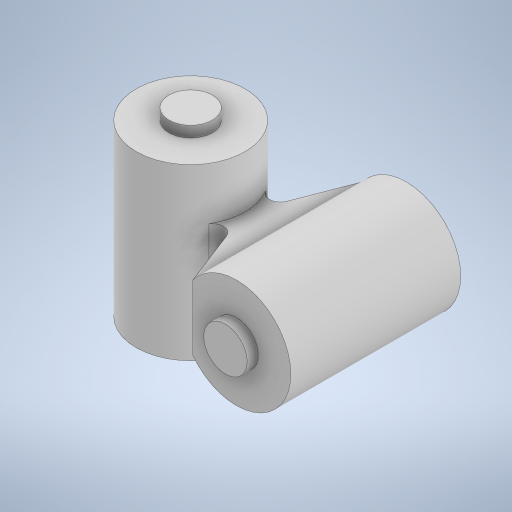
# Autodesk Inventor part: Arm 4 v0.1
Saved by Autodesk Inventor 2023 (Build 270158000, 158)
## iProperties
Created: 2024-06-24
Part Number: Arm 4 v0.1
Material: Generic
Document SubType Name: Modeling
Designer: Swoby
Density: 1 g/cm^3
Appearance: Default
Author: Swoby
Autodesk Inventor part; units mm, degrees
ref_plane "YZ Plane" through (0, 0, 0) normal (1, 0, 0) x (0, 1, 0)
ref_plane "XZ Plane" through (0, 0, 0) normal (0, 1, 0) x (-1, 0, 0)
ref_plane "XY Plane" through (0, 0, 0) normal (0, 0, 1) x (1, 0, 0)
sketch "Sketch1" plane through (0, 0, 0) normal (0, 0, 1) x (1, 0, 0)
  circle A0 centre (0, 0) radius 25
  circle A1 centre (0, 0) radius 10
  line L0 (-60, 15) -> (-20, 15)
  line L1 (-20, 15) -> (-20, -15)
  line L2 (-20, -15) -> (-60, -15)
  line L3 (-60, -15) -> (-60, 15)
  point P0 (-40, -15)
  point P1 (-20, -15)
  dimension "d0" = 50
  dimension "d1" = 20
  dimension "d2" = 30
  dimension "d3" = 15
  dimension "d4" = 40
  constraints: 8 end point, 2 coincident, 2 parallel, 1 centre point, 1 horizontal, 1 midpoint, 1 perpendicular, 3 other
  measures "d1" diameter of A1
  measures "d2" distance from line of point (-40, -15) L0
  measures "d3" distance from line of L0 point (0, 0)
  measures "d4" distance of L0.start L0.end
extrude "Extrusion1" add sketch "Sketch1" along normal mid plane 78 contours A0 L1 | L1 A0 | A0 L2 L3 L0 | A1
sketch "Sketch2" plane through (0, 0, 0) normal (0, 0, 1) x (1, 0, 0)
  circle A0 centre (0, 0) radius 10
  dimension "d7" = 20
  constraints: 1 centre point, 1 coincident
  measures "d7" diameter of A0
extrude "Extrusion2" add sketch "Sketch2" along normal mid plane 88
sketch "Sketch3" plane through (0, 0, 0) normal (0, 1, 0) x (-1, 0, 0)
  circle A0 centre (60, 0) radius 25
  line L0 (20, -39) -> (20, 39) construction
  line L1 (60, 39) -> (60, -39) projected
  line L2 (-25, -39) -> (20, -39) projected
  line L3 (20, 39) -> (-25, 39) projected
  line L4 (0, 0) -> (60, 0) construction
  line L5 (35, 0) -> (20, -39)
  line L6 (35, 0) -> (20, 39)
  arc A1 (38.6367, -12.9849) -> (29.6973, -13.787) centre (34.364, -15.5819) ccw
  arc A2 (29.6973, 13.787) -> (38.6367, 12.9849) centre (34.364, 15.5819) ccw
  line L7 (60, 39) -> (20, 39) projected
  line L8 (60, 25) -> (60, 39)
  line L9 (60, -39) -> (60, -25)
  line L10 (20, -39) -> (20, 39) projected
  line L11 (20, -39) -> (60, -39)
  dimension "d10" = 50
  dimension "d11" = 60
  dimension "d14" = 10
  dimension "d15" = 10
  constraints: 12 end point, 9 point on circle, 5 point on line, 4 tangent, 3 centre point, 2 perpendicular, 1 vertical
  measures "d10" diameter of A0
  measures "d11" distance of L4.end L4.start
  measures "d14" diameter of A1
  measures "d15" diameter of A2
extrude "Extrusion3" add sketch "Sketch3" along normal mid plane 78 contours A0 L1 | L1 A0
extrude "Extrusion4" cut sketch "Sketch3" along normal through all both and the other way through all contours A0 A2 L6 L7 L1 | L1 L11 L5 A1 A0
sketch "Sketch4" plane through (0, 0, 0) normal (0, 1, 0) x (-1, 0, 0)
  circle A0 centre (60, 0) radius 25 projected
  circle A1 centre (60, 0) radius 10
  point P0 (0, 0)
  dimension "d20" = 20
  constraints: 1 centre point, 1 coincident
  measures "d20" diameter of A1
extrude "Extrusion5" add sketch "Sketch4" along normal mid plane 88 contours A1
equation "\"d3\" = 0.5 * d2"
body "Solid1"
